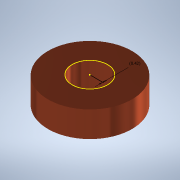
# Autodesk Inventor part: cilindro 1
Saved by Autodesk Inventor 2020 (Build 240168000, 168)
## iProperties
Created: 2015-10-12
Part Number: cilindro 1
Material: Copper
Document SubType Name: Modeling
Designer: Vaca
Density: 8.94 g/cm^3
Appearance: Copper - Satin
Author: Vaca
Autodesk Inventor part; units mm, degrees
ref_plane "YZ Plane" through (0, 0, 0) normal (1, 0, 0) x (0, 1, 0)
ref_plane "XZ Plane" through (0, 0, 0) normal (0, 1, 0) x (-1, 0, 0)
ref_plane "XY Plane" through (0, 0, 0) normal (0, 0, 1) x (1, 0, 0)
sketch "Sketch1" plane through (0, 0, 0) normal (0, 1, 0) x (-1, 0, 0)
  circle A0 centre (0, 0) radius 47.5
  constraints: 4 coincident, 1 centre point
extrude "Extrusion1" add sketch "Sketch1" along normal blind 29.1
sketch "Boceto3" plane through (0, 29.1, 0) normal (0, 1, 0) x (1, 0, 0)
  point P0 (-0.7708, 0.4202)
hole "Hole3" at (-0.7708, 29.1, -0.4202) direction (0, -1, 0) diameter 40 end through all
sketch "Sketch2" plane through (0, 29.1, 0) normal (0, 1, 0) x (1, 0, 0)
  circle A0 centre (-0.7708, 0.4202) radius 20 projected
  point P0 (0, 0)
  dimension "d34" = 0.42
body "Solid1"
